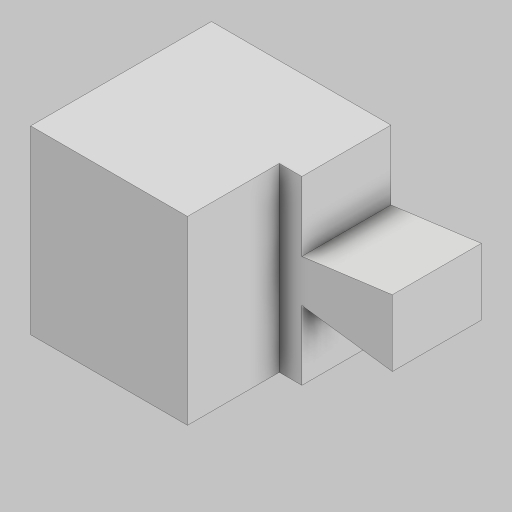
# Autodesk Inventor part: Macho
Saved by Autodesk Inventor 2023 (Build 270158000, 158)
## iProperties
Created: 2026-02-22
Part Number: Macho
Material: Genérico
Document SubType Name: Modeling
Designer: MARTIN MAESTRE
Density: 1 g/cm^3
Appearance: Valor por defecto
Author: MARTIN MAESTRE
Autodesk Inventor part; units mm, degrees
ref_plane "YZ Plane" through (0, 0, 0) normal (1, 0, 0) x (0, 1, 0)
ref_plane "XZ Plane" through (0, 0, 0) normal (0, 1, 0) x (-1, 0, 0)
ref_plane "XY Plane" through (0, 0, 0) normal (0, 0, 1) x (1, 0, 0)
sketch "Boceto1" plane through (0, 0, 0) normal (0, 0, 1) x (1, 0, 0)
  line L0 (0, 0) -> (0, 40)
  line L1 (0, 40) -> (39.7, 40)
  line L2 (0, 0) -> (39.7, 0)
  line L3 (39.7, 0) -> (39.7, 15.3)
  line L4 (39.7, 40) -> (39.7, 24.7)
  line L5 (39.7, 0) -> (59.7, 0) construction
  line L6 (39.7, 40) -> (59.7, 40) construction
  line L7 (59.7, 40) -> (59.7, 27.35) construction
  line L8 (59.7, 0) -> (59.7, 12.65) construction
  line L9 (39.7, 24.7) -> (59.7, 27.35)
  line L10 (39.7, 15.3) -> (59.7, 12.65)
  line L11 (59.7, 12.65) -> (59.7, 27.35)
  dimension "d0" = 40
  dimension "d1" = 39.7
  dimension "d2" = 39.7
  dimension "d3" = 15.3
  dimension "d4" = 15.3
  dimension "d5" = 20
  dimension "d6" = 20
  dimension "d7" = 12.65
  dimension "d8" = 12.65
  constraints: 24 end point, 5 vertical, 4 horizontal
  measures "d0" distance of L0.start L0.end
  measures "d1" distance of L0.end L1.end
  measures "d2" distance of L0.start L2.end
  measures "d3" distance of L2.end L3.end
  measures "d4" distance of L1.end L4.end
  measures "d5" distance of L2.end L5.end
  measures "d6" distance of L1.end L6.end
  measures "d7" distance of L6.end L7.end
  measures "d8" distance of L5.end L8.end
extrude "Extrusión1" add sketch "Boceto1" along normal blind 40
sketch "Boceto2" plane through (0, 0, 40) normal (0, 0, 1) x (1, 0, 0)
  line L0 (0, 0) -> (34.7, 0)
  line L1 (0, 0) -> (39.7, 0) projected
  line L2 (34.7, 0) -> (59.7, 0)
  line L3 (59.7, 0) -> (59.7, 40)
  line L4 (59.7, 40) -> (34.7, 40)
  line L5 (39.7, 40) -> (0, 40) projected
  line L6 (34.7, 0) -> (34.7, 40)
  dimension "d11" = 34.7
  dimension "d12" = 25
  dimension "d13" = 40
  dimension "d14" = 25
  constraints: 10 end point, 2 point on line, 1 horizontal, 1 perpendicular
  measures "d11" distance of L0.start L0.end
  measures "d12" distance of L0.end L2.end
  measures "d13" distance of L2.end L3.end
  measures "d14" distance of L3.end L4.end
extrude "Extrusión2" cut sketch "Boceto2" against normal blind 20.3
